# Autodesk Inventor part: Disc Cam
Saved by Autodesk Inventor 2015 (Build 190159000, 159)
## iProperties
Created: 2015-04-16
Part Number: Disc Cam
Material: Stainless Steel, Austenitic
Document SubType Name: Modeling
Designer: WASHHSST
Manufacturer: Standard
Standards Organization: Custom
Density: 1 g/cm^3
Appearance: Steel
CustomPartVersion: 1
Author: WASHHSST
Autodesk Inventor part; units mm, degrees
ref_plane "YZ Plane" through (0, 0, 0) normal (1, 0, 0) x (0, 1, 0)
ref_plane "XZ Plane" through (0, 0, 0) normal (0, 1, 0) x (-1, 0, 0)
ref_plane "XY Plane" through (0, 0, 0) normal (0, 0, 1) x (1, 0, 0)
sketch "Main Sketch" plane through (0, 0, 0) normal (0, 0, 1) x (1, 0, 0)
  spline S0 degree 5 poles (0, 101.6) (2.5662, 101.6) (6.848, 101.4663) (13.2705, 100.9373) (21.7896, 99.6326) (32.2479, 97.081) (42.0572, 93.8599) (51.9524, 89.7014) (61.458, 84.7582) (70.4932, 79.0142) (78.943, 72.4401) (86.6699, 64.9731) (93.5429, 56.5968) (99.423, 47.3458) (104.1804, 37.3252) (107.7295, 26.638) (109.992, 15.5266) (111.0324, 3.9841) (110.7926, -7.4151) (109.1117, -18.8871) (106.0795, -30.067) (101.7163, -40.8584) (96.1151, -51.0643) (89.3748, -60.5562) (81.6241, -69.2045) (73.0033, -76.9152) (63.6592, -83.6193) (53.7426, -89.2751) (43.3886, -93.8679) (32.7475, -97.3943) (21.9025, -99.8859) (11.0397, -101.3413) (0.0606, -101.8598) (-10.5581, -101.34) (-21.1733, -99.6539) (-31.4719, -96.8964) (-41.4403, -93.0702) (-50.9384, -88.2301) (-59.8834, -82.4216) (-68.1701, -75.7109) (-75.7109, -68.1703) (-82.4218, -59.883) (-88.2298, -50.9395) (-93.071, -41.4379) (-96.8926, -31.4823) (-99.6526, -21.1818) (-101.3208, -10.6492) (-101.8789, 0) (-101.3208, 10.6493) (-99.6527, 21.1818) (-96.8926, 31.4823) (-93.0711, 41.4379) (-88.2298, 50.9395) (-82.4218, 59.8829) (-75.7108, 68.1703) (-68.1703, 75.7108) (-59.883, 82.4218) (-50.9393, 88.2297) (-41.4383, 93.0712) (-31.8797, 96.7394) (-21.5993, 99.5536) (-13.1759, 100.9303) (-6.8113, 101.4672) (-2.5556, 101.6) (0, 101.6) knots 0 0 0 0 0 0 0.019853 0.033098 0.049652 0.066205 0.082745 0.099268 0.11578 0.132298 0.148848 0.165457 0.182153 0.198956 0.215874 0.232874 0.249943 0.267064 0.284218 0.301387 0.318584 0.335794 0.353001 0.370189 0.387344 0.404451 0.421499 0.438478 0.455383 0.472212 0.488938 0.505579 0.522149 0.538665 0.555141 0.571617 0.588094 0.60457 0.621046 0.637522 0.653999 0.670475 0.686951 0.703427 0.719904 0.73638 0.752856 0.769332 0.785809 0.802285 0.818761 0.835237 0.851714 0.86819 0.884666 0.901142 0.917619 0.934095 0.950571 0.967047 0.980228 1 1 1 1 1 1
  point P0 (21.3135, 99.4946)
  point P1 (31.7845, 97.0009)
  point P2 (41.9969, 93.6512)
  point P3 (51.8777, 89.4943)
  point P4 (61.3554, 84.5492)
  point P5 (70.3444, 78.8083)
  point P6 (78.7313, 72.2447)
  point P7 (86.3959, 64.8125)
  point P8 (93.2176, 56.486)
  point P9 (99.0655, 47.2934)
  point P10 (103.8158, 37.3152)
  point P11 (107.3696, 26.676)
  point P12 (109.6693, 15.5317)
  point P13 (110.7099, 4.0511)
  point P14 (110.4381, -7.3812)
  point P15 (108.7828, -18.7699)
  point P16 (105.7591, -29.9337)
  point P17 (101.4148, -40.6953)
  point P18 (95.8283, -50.889)
  point P19 (89.1046, -60.3674)
  point P20 (81.3702, -69.0065)
  point P21 (72.7658, -76.709)
  point P22 (63.4399, -83.4061)
  point P23 (53.5408, -89.0561)
  point P24 (43.2109, -93.6422)
  point P25 (32.582, -97.1675)
  point P26 (21.7714, -99.6502)
  point P27 (10.8815, -101.1176)
  point P28 (0, -101.6)
  point P29 (-10.6201, -101.0434)
  point P30 (-21.1238, -99.3798)
  point P31 (-31.3961, -96.6273)
  point P32 (-41.3244, -92.8162)
  point P33 (-50.8, -87.9882)
  point P34 (-59.719, -82.1961)
  point P35 (-67.9837, -75.5035)
  point P36 (-75.5035, -67.9837)
  point P37 (-82.1961, -59.719)
  point P38 (-87.9882, -50.8)
  point P39 (-92.8162, -41.3244)
  point P40 (-96.6273, -31.3961)
  point P41 (-99.3798, -21.1238)
  point P42 (-101.0434, -10.6201)
  point P43 (-101.6, 0)
  point P44 (-101.0434, 10.6201)
  point P45 (-99.3798, 21.1238)
  point P46 (-96.6273, 31.3961)
  point P47 (-92.8162, 41.3244)
  point P48 (-87.9882, 50.8)
  point P49 (-82.1961, 59.719)
  point P50 (-75.5035, 67.9837)
  point P51 (-67.9837, 75.5035)
  point P52 (-59.719, 82.1961)
  point P53 (-50.8, 87.9882)
  point P54 (-41.3244, 92.8162)
  point P55 (-31.3961, 96.6273)
  point P56 (-21.1238, 99.3798)
  point P57 (-10.6201, 101.0434)
  constraints: 60 other
extrude "Cam" add sketch "Main Sketch" along normal blind 12.7
body "Solid1"
